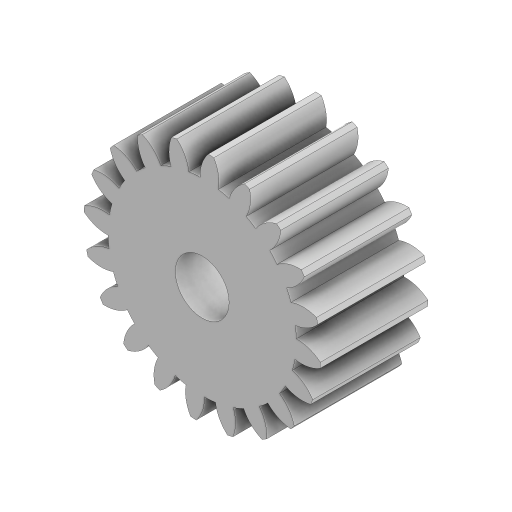
# Autodesk Inventor part: PLANETARIO SOL
Saved by Autodesk Inventor 2024 (Build 280153000, 153)
## iProperties
Created: 2024-06-18
Part Number: PLANETARIO SOL
Material: Generic
Document SubType Name: Modeling
Designer: Jhuliams
Density: 1 g/cm^3
Appearance: Default
Author: Jhuliams
Autodesk Inventor part; units mm, degrees
ref_plane "YZ Plane" through (0, 0, 0) normal (1, 0, 0) x (0, 1, 0)
ref_plane "XZ Plane" through (0, 0, 0) normal (0, 1, 0) x (-1, 0, 0)
ref_plane "XY Plane" through (0, 0, 0) normal (0, 0, 1) x (1, 0, 0)
sketch "Sketch1" plane through (0, 0, 0) normal (0, 0, 1) x (1, 0, 0)
  arc A0 (10.947, -1.0781) -> (10.9857, -0.5614) centre (0, 0) ccw
  circle A1 centre (0, 0) radius 8.75
  line L0 (0, 0) -> (18.5832, 0) construction
  arc A2 (10.9857, -0.5614) -> (8.7477, 0.2024) centre (8.8444, -3.175) ccw
  line L1 (0, 0) -> (16.1968, 0) construction
  line L2 (0, 0) -> (16.1894, 0) construction
  arc A3 (8.6204, -1.5007) -> (10.947, -1.0781) centre (9.2181, 1.8248) ccw
  arc A4 (10.7444, 2.3575) -> (10.6215, 2.8609) centre (0, 0) ccw
  arc A5 (10.6215, 2.8609) -> (8.257, 2.8956) centre (9.3926, -0.2865) ccw
  arc A6 (8.6622, 1.2366) -> (10.7444, 2.3575) centre (8.2031, 4.584) ccw
  arc A7 (9.49, 5.5623) -> (9.2176, 6.003) centre (0, 0) ccw
  arc A8 (9.2176, 6.003) -> (6.958, 5.3055) centre (9.0215, 2.63) ccw
  arc A9 (7.8561, 3.8529) -> (9.49, 5.5623) centre (6.385, 6.8946) ccw
  arc A10 (7.3067, 8.2226) -> (6.9114, 8.5576) centre (0, 0) ccw
  arc A11 (6.9114, 8.5576) -> (4.978, 7.196) centre (7.7672, 5.289) ccw
  arc A12 (6.281, 6.0919) -> (7.3067, 8.2226) centre (3.942, 8.5302) ccw
  arc A13 (4.4082, 10.0781) -> (3.9287, 10.2745) centre (0, 0) ccw
  arc A14 (3.9287, 10.2745) -> (2.5107, 8.3821) centre (5.7527, 7.4304) ccw
  arc A15 (4.0911, 7.7347) -> (4.4082, 10.0781) centre (1.1131, 9.3309) ccw
  arc A16 (1.0781, 10.947) -> (0.5614, 10.9857) centre (0, 0) ccw
  arc A17 (0.5614, 10.9857) -> (-0.2024, 8.7477) centre (3.175, 8.8444) ccw
  arc A18 (1.5007, 8.6204) -> (1.0781, 10.947) centre (-1.8248, 9.2181) ccw
  arc A19 (-2.3575, 10.7444) -> (-2.8609, 10.6215) centre (0, 0) ccw
  arc A20 (-2.8609, 10.6215) -> (-2.8956, 8.257) centre (0.2865, 9.3926) ccw
  arc A21 (-1.2366, 8.6622) -> (-2.3575, 10.7444) centre (-4.584, 8.2031) ccw
  arc A22 (-5.5623, 9.49) -> (-6.003, 9.2176) centre (0, 0) ccw
  arc A23 (-6.003, 9.2176) -> (-5.3055, 6.958) centre (-2.63, 9.0215) ccw
  arc A24 (-3.8529, 7.8561) -> (-5.5623, 9.49) centre (-6.8946, 6.385) ccw
  arc A25 (-8.2226, 7.3067) -> (-8.5576, 6.9114) centre (0, 0) ccw
  arc A26 (-8.5576, 6.9114) -> (-7.196, 4.978) centre (-5.289, 7.7672) ccw
  arc A27 (-6.0919, 6.281) -> (-8.2226, 7.3067) centre (-8.5302, 3.942) ccw
  arc A28 (-10.0781, 4.4082) -> (-10.2745, 3.9287) centre (0, 0) ccw
  arc A29 (-10.2745, 3.9287) -> (-8.3821, 2.5107) centre (-7.4304, 5.7527) ccw
  arc A30 (-7.7347, 4.0911) -> (-10.0781, 4.4082) centre (-9.3309, 1.1131) ccw
  arc A31 (-10.947, 1.0781) -> (-10.9857, 0.5614) centre (0, 0) ccw
  arc A32 (-10.9857, 0.5614) -> (-8.7477, -0.2024) centre (-8.8444, 3.175) ccw
  arc A33 (-8.6204, 1.5007) -> (-10.947, 1.0781) centre (-9.2181, -1.8248) ccw
  arc A34 (-10.7444, -2.3575) -> (-10.6215, -2.8609) centre (0, 0) ccw
  arc A35 (-10.6215, -2.8609) -> (-8.257, -2.8956) centre (-9.3926, 0.2865) ccw
  arc A36 (-8.6622, -1.2366) -> (-10.7444, -2.3575) centre (-8.2031, -4.584) ccw
  arc A37 (-9.49, -5.5623) -> (-9.2176, -6.003) centre (0, 0) ccw
  arc A38 (-9.2176, -6.003) -> (-6.958, -5.3055) centre (-9.0215, -2.63) ccw
  arc A39 (-7.8561, -3.8529) -> (-9.49, -5.5623) centre (-6.385, -6.8946) ccw
  arc A40 (-7.3067, -8.2226) -> (-6.9114, -8.5576) centre (0, 0) ccw
  arc A41 (-6.9114, -8.5576) -> (-4.978, -7.196) centre (-7.7672, -5.289) ccw
  arc A42 (-6.281, -6.0919) -> (-7.3067, -8.2226) centre (-3.942, -8.5302) ccw
  arc A43 (-4.4082, -10.0781) -> (-3.9287, -10.2745) centre (0, 0) ccw
  arc A44 (-3.9287, -10.2745) -> (-2.5107, -8.3821) centre (-5.7527, -7.4304) ccw
  arc A45 (-4.0911, -7.7347) -> (-4.4082, -10.0781) centre (-1.1131, -9.3309) ccw
  arc A46 (-1.0781, -10.947) -> (-0.5614, -10.9857) centre (0, 0) ccw
  arc A47 (-0.5614, -10.9857) -> (0.2024, -8.7477) centre (-3.175, -8.8444) ccw
  arc A48 (-1.5007, -8.6204) -> (-1.0781, -10.947) centre (1.8248, -9.2181) ccw
  arc A49 (2.3575, -10.7444) -> (2.8609, -10.6215) centre (0, 0) ccw
  arc A50 (2.8609, -10.6215) -> (2.8956, -8.257) centre (-0.2865, -9.3926) ccw
  arc A51 (1.2366, -8.6622) -> (2.3575, -10.7444) centre (4.584, -8.2031) ccw
  arc A52 (5.5623, -9.49) -> (6.003, -9.2176) centre (0, 0) ccw
  arc A53 (6.003, -9.2176) -> (5.3055, -6.958) centre (2.63, -9.0215) ccw
  arc A54 (3.8529, -7.8561) -> (5.5623, -9.49) centre (6.8946, -6.385) ccw
  arc A55 (8.2226, -7.3067) -> (8.5576, -6.9114) centre (0, 0) ccw
  arc A56 (8.5576, -6.9114) -> (7.196, -4.978) centre (5.289, -7.7672) ccw
  arc A57 (6.0919, -6.281) -> (8.2226, -7.3067) centre (8.5302, -3.942) ccw
  arc A58 (10.0781, -4.4082) -> (10.2745, -3.9287) centre (0, 0) ccw
  arc A59 (10.2745, -3.9287) -> (8.3821, -2.5107) centre (7.4304, -5.7527) ccw
  arc A60 (7.7347, -4.0911) -> (10.0781, -4.4082) centre (9.3309, -1.1131) ccw
  circle A61 centre (0, 0) radius 2.5
  point P0 (-0.2024, 8.7477)
  point P1 (-1.2366, 8.6622)
  point P2 (-2.8956, 8.257)
  point P3 (-3.8529, 7.8561)
  point P4 (-5.3055, 6.958)
  point P5 (-8.7477, -0.2024)
  point P6 (-8.257, -2.8956)
  point P7 (-7.8561, -3.8529)
  point P8 (-6.958, -5.3055)
  point P9 (-4.0911, -7.7347)
  point P10 (-2.5107, -8.3821)
  point P11 (0.2024, -8.7477)
  point P12 (1.2366, -8.6622)
  point P13 (2.8956, -8.257)
  point P14 (3.8529, -7.8561)
  point P15 (7.196, -4.978)
  point P16 (7.7347, -4.0911)
  point P17 (8.3821, -2.5107)
  point P18 (8.6622, 1.2366)
  point P19 (8.257, 2.8956)
  point P20 (7.8561, 3.8529)
  point P21 (6.958, 5.3055)
  point P22 (4.978, 7.196)
  point P23 (4.0911, 7.7347)
  point P24 (2.5107, 8.3821)
  dimension "d2" = 17.5
  dimension "d1" = 22
  dimension "d8" = 360
  dimension "d10" = 5
  constraints: 120 point on circle, 61 centre point, 6 end point, 3 horizontal, 2 coincident, 204 other
  measures "d1" diameter of A0
  measures "d10" diameter of A61
extrude "Extrusion1" add sketch "Sketch1" along normal blind 10
body "Solid1"
